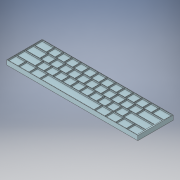
# Autodesk Inventor part: keyboard-base_standard
Saved by Autodesk Inventor 2016 (Build 200138000, 138)
## iProperties
Created: 2016-12-08
Part Number: keyboard-base_standard
Material: Generic
Document SubType Name: Modeling
Designer: Cemra JC
Density: 1 g/cm^3
Appearance: Default
Author: Cemra JC
Autodesk Inventor part; units mm, degrees
ref_plane "YZ Plane" through (0, 0, 0) normal (1, 0, 0) x (0, 1, 0)
ref_plane "XZ Plane" through (0, 0, 0) normal (0, 1, 0) x (-1, 0, 0)
ref_plane "XY Plane" through (0, 0, 0) normal (0, 0, 1) x (1, 0, 0)
sketch "Keyboard Backplane" plane through (0, 0, 0) normal (0, 1, 0) x (-1, 0, 0)
  line L0 (138.75, 37.5) -> (-138.75, 37.5)
  line L1 (-138.75, 37.5) -> (-138.75, -37.5)
  line L2 (-138.75, -37.5) -> (138.75, -37.5)
  line L3 (138.75, -37.5) -> (138.75, 37.5)
  line L4 (138.75, 37.5) -> (-138.75, -37.5) construction
  line L5 (-138.75, 37.5) -> (138.75, -37.5) construction
  point P0 (0, 0)
  point P1 (0, 0)
  dimension "d0" = 75
  dimension "d1" = 277.5
  constraints: 12 end point, 2 parallel, 1 coincident, 1 horizontal, 1 midpoint, 1 perpendicular
  measures "d0" distance of L0.end L1.end
  measures "d1" distance of L1.end L2.end
extrude "Keyboard Backplane Body" add sketch "Keyboard Backplane" along normal blind 10
sketch "KeyCap Outlines" plane through (0, 10, 0) normal (0, 1, 0) x (1, 0, 0)
  line L0 (-137.75, 36.5) -> (-111.5, 36.5)
  line L1 (-111.5, 36.5) -> (-111.5, 19)
  line L2 (-111.5, 19) -> (-137.75, 19)
  line L3 (-137.75, 19) -> (-137.75, 36.5)
  line L4 (-138.75, -37.5) -> (138.75, -37.5) projected
  line L5 (138.75, -37.5) -> (138.75, 37.5) projected
  line L6 (138.75, 37.5) -> (-138.75, 37.5) projected
  line L7 (-138.75, 37.5) -> (-138.75, -37.5) projected
  line L8 (-110.5, 19) -> (-93, 19)
  line L9 (-93, 19) -> (-93, 36.5)
  line L10 (-93, 36.5) -> (-110.5, 36.5)
  line L11 (-110.5, 36.5) -> (-110.5, 19)
  line L12 (-92, 19) -> (-74.5, 19)
  line L13 (-74.5, 19) -> (-74.5, 36.5)
  line L14 (-74.5, 36.5) -> (-92, 36.5)
  line L15 (-92, 36.5) -> (-92, 19)
  line L16 (-73.5, 19) -> (-56, 19)
  line L17 (-56, 19) -> (-56, 36.5)
  line L18 (-56, 36.5) -> (-73.5, 36.5)
  line L19 (-73.5, 36.5) -> (-73.5, 19)
  line L20 (-55, 19) -> (-37.5, 19)
  line L21 (-37.5, 19) -> (-37.5, 36.5)
  line L22 (-37.5, 36.5) -> (-55, 36.5)
  line L23 (-55, 36.5) -> (-55, 19)
  line L24 (-36.5, 19) -> (-19, 19)
  line L25 (-19, 19) -> (-19, 36.5)
  line L26 (-19, 36.5) -> (-36.5, 36.5)
  line L27 (-36.5, 36.5) -> (-36.5, 19)
  line L28 (-18, 19) -> (-0.5, 19)
  line L29 (-0.5, 19) -> (-0.5, 36.5)
  line L30 (-0.5, 36.5) -> (-18, 36.5)
  line L31 (-18, 36.5) -> (-18, 19)
  line L32 (0.5, 19) -> (18, 19)
  line L33 (18, 19) -> (18, 36.5)
  line L34 (18, 36.5) -> (0.5, 36.5)
  line L35 (0.5, 36.5) -> (0.5, 19)
  line L36 (19, 19) -> (36.5, 19)
  line L37 (36.5, 19) -> (36.5, 36.5)
  line L38 (36.5, 36.5) -> (19, 36.5)
  line L39 (19, 36.5) -> (19, 19)
  line L40 (37.5, 19) -> (55, 19)
  line L41 (55, 19) -> (55, 36.5)
  line L42 (55, 36.5) -> (37.5, 36.5)
  line L43 (37.5, 36.5) -> (37.5, 19)
  line L44 (56, 19) -> (73.5, 19)
  line L45 (73.5, 19) -> (73.5, 36.5)
  line L46 (73.5, 36.5) -> (56, 36.5)
  line L47 (56, 36.5) -> (56, 19)
  line L48 (74.5, 19) -> (92, 19)
  line L49 (92, 19) -> (92, 36.5)
  line L50 (92, 36.5) -> (74.5, 36.5)
  line L51 (74.5, 36.5) -> (74.5, 19)
  line L52 (93, 19) -> (110.5, 19)
  line L53 (110.5, 19) -> (110.5, 36.5)
  line L54 (110.5, 36.5) -> (93, 36.5)
  line L55 (93, 36.5) -> (93, 19)
  line L56 (111.5, 36.5) -> (137.75, 36.5)
  line L57 (137.75, 36.5) -> (137.75, 19)
  line L58 (137.75, 19) -> (111.5, 19)
  line L59 (111.5, 19) -> (111.5, 36.5)
  line L60 (-137.75, 18) -> (-107.125, 18)
  line L61 (-107.125, 18) -> (-107.125, 0.5)
  line L62 (-107.125, 0.5) -> (-137.75, 0.5)
  line L63 (-137.75, 0.5) -> (-137.75, 18)
  line L64 (-106.125, 0.5) -> (-88.625, 0.5)
  line L65 (-88.625, 0.5) -> (-88.625, 18)
  line L66 (-88.625, 18) -> (-106.125, 18)
  line L67 (-106.125, 18) -> (-106.125, 0.5)
  line L68 (-70.125, 0.5) -> (-70.125, 18)
  line L69 (-70.125, 18) -> (-87.625, 18)
  line L70 (-87.625, 18) -> (-87.625, 0.5)
  line L71 (-87.625, 0.5) -> (-70.125, 0.5)
  line L72 (-51.625, 0.5) -> (-51.625, 18)
  line L73 (-51.625, 18) -> (-69.125, 18)
  line L74 (-69.125, 18) -> (-69.125, 0.5)
  line L75 (-69.125, 0.5) -> (-51.625, 0.5)
  line L76 (-33.125, 0.5) -> (-33.125, 18)
  line L77 (-33.125, 18) -> (-50.625, 18)
  line L78 (-50.625, 18) -> (-50.625, 0.5)
  line L79 (-50.625, 0.5) -> (-33.125, 0.5)
  line L80 (-14.625, 0.5) -> (-14.625, 18)
  line L81 (-14.625, 18) -> (-32.125, 18)
  line L82 (-32.125, 18) -> (-32.125, 0.5)
  line L83 (-32.125, 0.5) -> (-14.625, 0.5)
  line L84 (3.875, 0.5) -> (3.875, 18)
  line L85 (3.875, 18) -> (-13.625, 18)
  line L86 (-13.625, 18) -> (-13.625, 0.5)
  line L87 (-13.625, 0.5) -> (3.875, 0.5)
  line L88 (22.375, 0.5) -> (22.375, 18)
  line L89 (22.375, 18) -> (4.875, 18)
  line L90 (4.875, 18) -> (4.875, 0.5)
  line L91 (4.875, 0.5) -> (22.375, 0.5)
  line L92 (40.875, 0.5) -> (40.875, 18)
  line L93 (40.875, 18) -> (23.375, 18)
  line L94 (23.375, 18) -> (23.375, 0.5)
  line L95 (23.375, 0.5) -> (40.875, 0.5)
  line L96 (59.375, 0.5) -> (59.375, 18)
  line L97 (59.375, 18) -> (41.875, 18)
  line L98 (41.875, 18) -> (41.875, 0.5)
  line L99 (41.875, 0.5) -> (59.375, 0.5)
  line L100 (77.875, 0.5) -> (77.875, 18)
  line L101 (77.875, 18) -> (60.375, 18)
  line L102 (60.375, 18) -> (60.375, 0.5)
  line L103 (60.375, 0.5) -> (77.875, 0.5)
  line L104 (96.375, 0.5) -> (96.375, 18)
  line L105 (96.375, 18) -> (78.875, 18)
  line L106 (78.875, 18) -> (78.875, 0.5)
  line L107 (78.875, 0.5) -> (96.375, 0.5)
  line L108 (97.375, 18) -> (136.75, 18)
  line L109 (136.75, 18) -> (136.75, 0.5)
  line L110 (136.75, 0.5) -> (97.375, 0.5)
  line L111 (97.375, 0.5) -> (97.375, 18)
  line L112 (-137.75, -0.5) -> (-98.375, -0.5)
  line L113 (-98.375, -0.5) -> (-98.375, -18)
  line L114 (-98.375, -18) -> (-137.75, -18)
  line L115 (-137.75, -18) -> (-137.75, -0.5)
  line L116 (-97.375, -0.5) -> (-79.875, -0.5)
  line L117 (-79.875, -0.5) -> (-79.875, -18)
  line L118 (-79.875, -18) -> (-97.375, -18)
  line L119 (-97.375, -18) -> (-97.375, -0.5)
  line L120 (-61.375, -18) -> (-78.875, -18)
  line L121 (-61.375, -0.5) -> (-61.375, -18)
  line L122 (-78.875, -18) -> (-78.875, -0.5)
  line L123 (-78.875, -0.5) -> (-61.375, -0.5)
  line L124 (-42.875, -18) -> (-60.375, -18)
  line L125 (-42.875, -0.5) -> (-42.875, -18)
  line L126 (-60.375, -18) -> (-60.375, -0.5)
  line L127 (-60.375, -0.5) -> (-42.875, -0.5)
  line L128 (-24.375, -18) -> (-41.875, -18)
  line L129 (-24.375, -0.5) -> (-24.375, -18)
  line L130 (-41.875, -18) -> (-41.875, -0.5)
  line L131 (-41.875, -0.5) -> (-24.375, -0.5)
  line L132 (-5.875, -18) -> (-23.375, -18)
  line L133 (-5.875, -0.5) -> (-5.875, -18)
  line L134 (-23.375, -18) -> (-23.375, -0.5)
  line L135 (-23.375, -0.5) -> (-5.875, -0.5)
  line L136 (12.625, -18) -> (-4.875, -18)
  line L137 (12.625, -0.5) -> (12.625, -18)
  line L138 (-4.875, -18) -> (-4.875, -0.5)
  line L139 (-4.875, -0.5) -> (12.625, -0.5)
  line L140 (31.125, -18) -> (13.625, -18)
  line L141 (31.125, -0.5) -> (31.125, -18)
  line L142 (13.625, -18) -> (13.625, -0.5)
  line L143 (13.625, -0.5) -> (31.125, -0.5)
  line L144 (49.625, -18) -> (32.125, -18)
  line L145 (49.625, -0.5) -> (49.625, -18)
  line L146 (32.125, -18) -> (32.125, -0.5)
  line L147 (32.125, -0.5) -> (49.625, -0.5)
  line L148 (68.125, -18) -> (50.625, -18)
  line L149 (68.125, -0.5) -> (68.125, -18)
  line L150 (50.625, -18) -> (50.625, -0.5)
  line L151 (50.625, -0.5) -> (68.125, -0.5)
  line L152 (86.625, -18) -> (69.125, -18)
  line L153 (86.625, -0.5) -> (86.625, -18)
  line L154 (69.125, -18) -> (69.125, -0.5)
  line L155 (69.125, -0.5) -> (86.625, -0.5)
  line L156 (87.625, -18) -> (135.75, -18)
  line L157 (135.75, -18) -> (135.75, -0.5)
  line L158 (135.75, -0.5) -> (87.625, -0.5)
  line L159 (87.625, -0.5) -> (87.625, -18)
  line L160 (-137.75, -36.5) -> (-115.875, -36.5)
  line L161 (-115.875, -36.5) -> (-115.875, -19)
  line L162 (-115.875, -19) -> (-137.75, -19)
  line L163 (-137.75, -19) -> (-137.75, -36.5)
  line L164 (-137.75, -36.5) -> (-115.875, -19) construction
  line L165 (-115.875, -36.5) -> (-137.75, -19) construction
  line L166 (-93, -36.5) -> (-93, -19)
  line L167 (-93, -19) -> (-114.875, -19)
  line L168 (-114.875, -19) -> (-114.875, -36.5)
  line L169 (-114.875, -36.5) -> (-93, -36.5)
  line L170 (-70.125, -36.5) -> (-70.125, -19)
  line L171 (-70.125, -19) -> (-92, -19)
  line L172 (-92, -19) -> (-92, -36.5)
  line L173 (-92, -36.5) -> (-70.125, -36.5)
  line L174 (-69.125, -19) -> (44.625, -19)
  line L175 (44.625, -19) -> (44.625, -36.5)
  line L176 (44.625, -36.5) -> (-69.125, -36.5)
  line L177 (-69.125, -36.5) -> (-69.125, -19)
  line L178 (45.625, -19) -> (67.5, -19)
  line L179 (67.5, -19) -> (67.5, -36.5)
  line L180 (67.5, -36.5) -> (45.625, -36.5)
  line L181 (45.625, -36.5) -> (45.625, -19)
  line L182 (90.375, -36.5) -> (68.5, -36.5)
  line L183 (68.5, -36.5) -> (68.5, -19)
  line L184 (68.5, -19) -> (90.375, -19)
  line L185 (90.375, -19) -> (90.375, -36.5)
  line L186 (113.25, -36.5) -> (91.375, -36.5)
  line L187 (91.375, -36.5) -> (91.375, -19)
  line L188 (91.375, -19) -> (113.25, -19)
  line L189 (113.25, -19) -> (113.25, -36.5)
  line L190 (136.125, -36.5) -> (114.25, -36.5)
  line L191 (114.25, -36.5) -> (114.25, -19)
  line L192 (114.25, -19) -> (136.125, -19)
  line L193 (136.125, -19) -> (136.125, -36.5)
  point P0 (0, 0)
  point P1 (-126.8125, -27.75)
  dimension "d4" = 26.25
  dimension "d5" = 17.5
  dimension "d6" = 1
  dimension "d7" = 1
  dimension "d8" = 17.5
  dimension "d9" = 17.5
  dimension "d10" = 1
  dimension "d11" = 1
  dimension "d14" = 18.5
  dimension "d19" = 26.25
  dimension "d20" = 17.5
  dimension "d21" = 1
  dimension "d22" = 1
  dimension "d23" = 17.5
  dimension "d24" = 30.625
  dimension "d25" = 1
  dimension "d26" = 1
  dimension "d27" = 17.5
  dimension "d28" = 17.5
  dimension "d29" = 1
  dimension "d30" = 1
  dimension "d33" = 18.5
  dimension "d38" = 17.5
  dimension "d39" = 39.375
  dimension "d40" = 1
  dimension "d41" = 1
  dimension "d42" = 17.5
  dimension "d43" = 39.375
  dimension "d44" = 1
  dimension "d45" = 1
  dimension "d46" = 17.5
  dimension "d47" = 17.5
  dimension "d48" = 1
  dimension "d49" = 1
  dimension "d52" = 18.5
  dimension "d57" = 17.5
  dimension "d58" = 48.125
  dimension "d59" = 1
  dimension "d60" = 1
  dimension "d63" = 21.875
  dimension "d64" = 17.5
  dimension "d65" = 1
  dimension "d66" = 1
  dimension "d69" = 22.875
  dimension "d74" = 113.75
  dimension "d75" = 17.5
  dimension "d76" = 1
  dimension "d77" = 1
  dimension "d78" = 21.875
  dimension "d79" = 17.5
  dimension "d80" = 1
  dimension "d81" = 1
  dimension "d84" = 22.875
  constraints: 380 end point, 24 parallel, 17 horizontal, 12 perpendicular, 5 collinear, 2 midpoint, 275 other
  measures "d4" distance of L1.end L2.end
  measures "d5" distance of L0.end L1.end
  measures "d6" distance between parallel lines of L6 L0
  measures "d7" distance between parallel lines of L7 L3
  measures "d8" distance of L10.end L9.end
  measures "d9" distance of L9.end L8.end
  measures "d10" distance between parallel lines of L6 L10
  measures "d11" distance between parallel lines of L1 L11
  measures "d14" distance of L8.start L12.start
  measures "d19" distance of L57.end L58.end
  measures "d20" distance of L56.end L57.end
  measures "d21" distance between parallel lines of L6 L56
  measures "d22" distance between parallel lines of L53 L59
  measures "d23" distance of L60.end L61.end
  measures "d24" distance of L61.end L62.end
  measures "d25" distance between parallel lines of L2 L60
  measures "d26" distance between parallel lines of L7 L63
  measures "d27" distance of L65.end L66.end
  measures "d28" distance of L64.end L65.end
  measures "d29" distance between parallel lines of L8 L66
  measures "d30" distance between parallel lines of L61 L67
  measures "d33" distance of L64.end L68.start
  measures "d38" distance of L108.end L109.end
  measures "d39" distance of L109.end L110.end
  measures "d40" distance between parallel lines of L104 L111
  measures "d41" distance between parallel lines of L58 L108
  measures "d42" distance of L112.end L113.end
  measures "d43" distance of L113.end L114.end
  measures "d44" distance between parallel lines of L7 L115
  measures "d45" distance between parallel lines of L62 L112
  measures "d46" distance of L116.end L117.end
  measures "d47" distance of L117.end L118.end
  measures "d48" distance between parallel lines of L113 L119
  measures "d49" distance between parallel lines of L64 L116
  measures "d52" distance of L117.end L120.start
  measures "d57" distance of L156.end L157.end
  measures "d58" distance of L156.start L156.end
  measures "d59" distance between parallel lines of L153 L159
  measures "d60" distance between parallel lines of L110 L158
  measures "d63" distance of L162.end L161.end
  measures "d64" distance of L161.end L160.end
  measures "d65" distance between parallel lines of L114 L162
  measures "d66" distance between parallel lines of L7 L163
  measures "d69" distance of L160.end L166.start
  measures "d74" distance of L175.end L176.end
  measures "d75" distance of L174.end L175.end
  measures "d76" distance between parallel lines of L170 L177
  measures "d77" distance between parallel lines of L120 L174
  measures "d78" distance of L179.end L180.end
  measures "d79" distance of L178.end L179.end
  measures "d80" distance between parallel lines of L144 L178
  measures "d81" distance between parallel lines of L175 L181
  measures "d84" distance of L179.end L182.start
extrude "Keycap Holes" cut sketch "KeyCap Outlines" against normal blind 3 contours L0 L1 L2 L3 | L11 L10 L9 L8 | L15 L14 L13 L12 | L19 L18 L17 L16 | L23 L22 L21 L20 | L27 L26 L25 L24 | L31 L30 L29 L28 | L35 L34 L33 L32 | L39 L38 L37 L36 | L43 L42 L41 L40 | L47 L46 L45 L44 | L51 L50 L49 L48 | L55 L54 L53 L52 | L56 L57 L58 L59 | L60 L61 L62 L63 | L67 L66 L65 L64 | L71 L70 L69 L68 | L75 L74 L73 L72 | L79 L78 L77 L76 | L83 L82 L81 L80 | L87 L86 L85 L84 | L91 L90 L89 L88 | L95 L94 L93 L92 | L99 L98 L97 L96 | L103 L102 L101 L100 | L107 L106 L105 L104 | L108 L109 L110 L111 | L112 L113 L114 L115 | L116 L117 L118 L119 | L120 L122 L123 L121 | L124 L126 L127 L125 | L128 L130 L131 L129 | L132 L134 L135 L133 | L136 L138 L139 L137 | L140 L142 L143 L141 | L144 L146 L147 L145 | L148 L150 L151 L149 | L152 L154 L155 L153 | L159 L158 L157 L156 | L163 L162 L161 L160 | L169 L168 L167 L166 | L173 L172 L171 L170 | L174 L175 L176 L177 | L178 L179 L180 L181 | L182 L183 L184 L185 | L186 L187 L188 L189 | L190 L191 L192 L193
equation "\"d0\" = b_height"
equation "\"d1\" = b_width"
equation "\"d4\" = b_tab"
equation "\"d5\" = k_width"
equation "\"d6\" = d7"
equation "\"d7\" = b_pad"
equation "\"d8\" = d5"
equation "\"d9\" = d5"
equation "\"d10\" = d6"
equation "\"d11\" = d7"
equation "\"d14\" = d8 + b_pad"
equation "\"d19\" = d4"
equation "\"d20\" = d5"
equation "\"d21\" = d7"
equation "\"d22\" = d7"
equation "\"d23\" = d5"
equation "\"d24\" = b_caps"
equation "\"d25\" = d7"
equation "\"d26\" = d7"
equation "\"d27\" = d5"
equation "\"d28\" = d5"
equation "\"d29\" = b_pad"
equation "\"d30\" = d29"
equation "\"d33\" = d27 + d7"
equation "\"d38\" = d5"
equation "\"d39\" = b_lshift"
equation "\"d40\" = d7"
equation "\"d41\" = d7"
equation "\"d42\" = d5"
equation "\"d43\" = d39"
equation "\"d44\" = d7"
equation "\"d45\" = d7"
equation "\"d46\" = d5"
equation "\"d47\" = d5"
equation "\"d48\" = d7"
equation "\"d49\" = d7"
equation "\"d52\" = d47 + d48"
equation "\"d57\" = d5"
equation "\"d58\" = b_rshift"
equation "\"d59\" = d7"
equation "\"d60\" = d7"
equation "\"d63\" = b_ctrl"
equation "\"d64\" = d5"
equation "\"d65\" = d7"
equation "\"d66\" = d7"
equation "\"d69\" = b_ctrl + b_pad"
equation "\"d74\" = b_space"
equation "\"d75\" = d5"
equation "\"d76\" = d7"
equation "\"d77\" = d7"
equation "\"d78\" = b_ctrl"
equation "\"d79\" = k_width"
equation "\"d80\" = d7"
equation "\"d81\" = d7"
equation "\"d84\" = b_ctrl + b_pad"
equation "\"k_width\" = 17.5"
equation "\"k_height\" = 16.5"
equation "\"k_taper1\" = 1.5"
equation "\"k_taper2\" = 0.5"
equation "\"k_radius\" = 6"
equation "\"k_wthick\" = 1.5"
equation "\"k_ribthick\" = 1.5"
equation "\"k_ribheight\" = 5"
equation "\"k_poleoff\" = 2.1875"
equation "\"k_poledia\" = 5.3"
equation "\"k_cmxw\" = 1.1"
equation "\"k_cmxl\" = 4.15"
equation "\"s_bwidth\" = 14.4"
equation "\"s_poleh\" = 3.6"
equation "\"s_polebw\" = 5.4"
equation "\"s_polebl\" = 7.45"
equation "\"b_pad\" = 1"
equation "\"b_tab\" = 26.25"
equation "\"b_caps\" = 30.625"
equation "\"b_lshift\" = 39.375"
equation "\"b_rshift\" = 48.125"
equation "\"b_ctrl\" = 21.875"
equation "\"b_space\" = 113.75"
equation "\"b_width\" = 277.5"
equation "\"b_height\" = 75"
equation "\"k_staper\" = 1"
equation "\"k_ltaper\" = 1.5"
equation "\"k_lradius\" = 6"
equation "\"k_sradius\" = 4"
equation "\"k_height_t\" = 16"
equation "\"k_taper_wide\" = 1.5"
equation "\"k_height_low\" = 15"
equation "\"k_taper_thin\" = 0.0001"
equation "\"k_shortening\" = 4.5"
equation "\"k_cmxd\" = 4"
body "Solid1"
